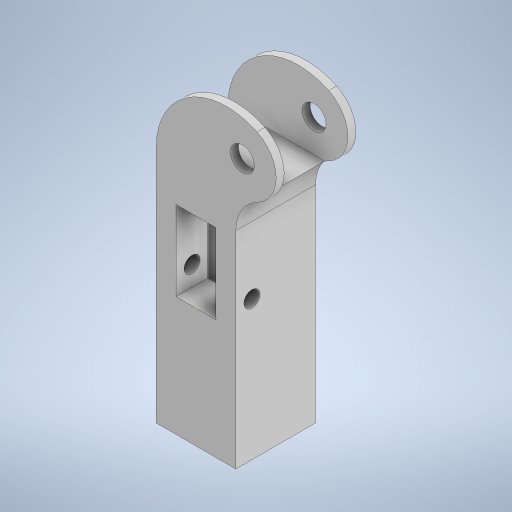
# Autodesk Inventor part: Unterstützen
Saved by Autodesk Inventor 2023 (Build 270158000, 158)
## iProperties
Created: 2024-02-02
Part Number: Unterstützen
Material: Generisch
Document SubType Name: Modeling
Designer: jefar
Density: 1 g/cm^3
Appearance: Vorgabe
Author: jefar
Autodesk Inventor part; units mm, degrees
ref_plane "YZ Plane" through (0, 0, 0) normal (1, 0, 0) x (0, 1, 0)
ref_plane "XZ Plane" through (0, 0, 0) normal (0, 1, 0) x (-1, 0, 0)
sketch "Skizze1" plane through (0, 0, 0) normal (0, 0, 1) x (1, 0, 0)
  line L0 (-1066.0722, 0) -> (1356.4088, 0) construction
  line L1 (0, -2329.2869) -> (0, 3475.7215) construction
  line L2 (500, 1091.469) -> (500, -1500)
  line L3 (500, -1500) -> (-500, -1500)
  line L4 (-500, -1500) -> (-500, 1500)
  line L5 (-500, 1500) -> (500, -1500) construction
  line L6 (500, 1500) -> (-500, -1500) construction
  arc A0 (765.6976, 2297.0927) -> (-500, 1500) centre (383.8395, 1500) ccw
  arc A1 (774.0795, 1537.5182) -> (765.6976, 2297.0927) centre (582.7661, 1915.2406) ccw
  circle A2 centre (582.7661, 1915.2406) radius 150
  arc A3 (774.0795, 1537.5182) -> (500, 1091.469) centre (1000, 1091.469) ccw
  point P0 (0, 0)
  dimension "d0" = 1000
  dimension "d1" = 3000
  dimension "d2" = 423.4087
  dimension "d3" = 300
  dimension "d5" = 500
  constraints: 10 end point, 7 point on circle, 4 centre point, 4 tangent, 2 midpoint, 1 coincident, 1 parallel, 1 point on line
  measures "d0" distance of L2.end L3.end
  measures "d1" distance of L6.start L2.end
  measures "d2" radius of A1
  measures "d3" diameter of A2
  measures "d5" radius of A3
extrude "Extrusion1" add sketch "Skizze1" along normal blind 1000
ref_plane "Arbeitsebene1" through (0, -1500, 0) normal (-1, 0, 0) x (0, 0, 1)
sketch "Skizze2" plane through (0, -1500, 0) normal (-1, 0, 0) x (0, 0, 1)
  line L0 (0, 3000) -> (1000, 3000) projected
  line L1 (100, 3000) -> (908.6027, 3000)
  line L2 (0, 3883.8395) -> (1000, 3883.8395) construction
  line L3 (100, 3000) -> (900, 3000)
  line L4 (900, 3000) -> (900, 3883.8395)
  line L5 (900, 3883.8395) -> (100, 3883.8395)
  line L6 (100, 3883.8395) -> (100, 3000)
  line L7 (1000, 3000) -> (1000, 3883.8395) construction
  point P0 (0, 1500)
  point P1 (1000, 3797.0927)
  dimension "d8" = 800
  dimension "d9" = 100
  constraints: 10 end point, 3 point on line, 2 parallel, 1 horizontal, 1 perpendicular
  measures "d8" distance of L5.end L4.end
  measures "d9" distance between parallel lines of L7 L4
extrude "Extrusion2" cut sketch "Skizze2" along normal mid plane 2500
sketch "Skizze3" plane through (0, 0, 1000) normal (0, 0, 1) x (1, 0, 0)
  point P0 (0, 0)
sketch "Skizze4" plane through (0, 0, 1000) normal (0, 0, 1) x (1, 0, 0)
  point P0 (0, 0)
sketch "Skizze5" plane through (0, 0, 1000) normal (0, 0, 1) x (1, 0, 0)
  line L0 (-500, 1500) -> (-500, -1500) construction
  line L1 (0, 0) -> (-250, 0)
  line L2 (-250, 0) -> (-250, 1000)
  line L3 (-250, 1000) -> (0, 1000)
  line L4 (0, 1000) -> (250, 1000)
  line L5 (250, 1000) -> (250, 0)
  line L6 (250, 0) -> (0, 0)
  line L7 (-250, 1000) -> (250, 1000)
  line L8 (250, 1000) -> (250, 0)
  line L9 (250, 0) -> (-250, 0)
  line L10 (-250, 0) -> (-250, 1000)
  dimension "d13" = 250
  dimension "d14" = 1000
  dimension "d15" = 250
  constraints: 20 end point, 4 parallel, 3 horizontal, 3 perpendicular, 1 point on line
  measures "d13" distance of L2.end L3.end
  measures "d14" distance of L1.end L2.end
  measures "d15" distance of L5.end L6.end
extrude "Extrusion3" cut sketch "Skizze5" against normal blind 400
sketch "Skizze6" plane through (-500, -1500, 0) normal (-1, 0, 0) x (0, 0, 1)
  point P0 (0, 1500)
sketch "Skizze7" plane through (-500, -1500, 0) normal (-1, 0, 0) x (0, 0, 1)
  point P0 (0, 1500)
sketch "Skizze8" plane through (-500, -1500, 0) normal (0, -1, 0) x (1, 0, 0)
  point P0 (500, 0)
sketch "Skizze9" plane through (-500, -1500, 0) normal (-1, 0, 0) x (0, 0, 1)
  line L0 (1000, 0) -> (800, 0)
  circle A0 centre (800, 1750) radius 100
  point P0 (0, 1500)
  constraints: 2 end point, 1 centre point, 1 horizontal
extrude "Extrusion4" cut sketch "Skizze9" against normal through all
sketch "Skizze10" plane through (0, 0, 1000) normal (0, 0, 1) x (1, 0, 0)
  point P0 (0, 0)
